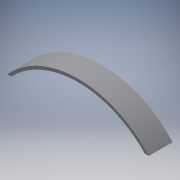
# Autodesk Inventor part: bumper
Saved by Autodesk Inventor 2016 (Build 200138000, 138)
## iProperties
Created: 2015-09-30
Part Number: bumper
Material: Generic
Document SubType Name: Modeling
Designer: Jesse Stevenson
Density: 1 g/cm^3
Appearance: Default
Author: Jesse Stevenson
Autodesk Inventor part; units mm, degrees
ref_plane "YZ Plane" through (0, 0, 0) normal (1, 0, 0) x (0, 1, 0)
ref_plane "XZ Plane" through (0, 0, 0) normal (0, 1, 0) x (-1, 0, 0)
ref_plane "XY Plane" through (0, 0, 0) normal (0, 0, 1) x (1, 0, 0)
sketch "Sketch1" plane through (0, 0, 0) normal (0, 0, 1) x (1, 0, 0)
  arc A0 (0, 0) -> (-150.9369, 0) centre (-75.4685, -68.0226) ccw
  arc A1 (-4.3319, 0) -> (-146.605, 0) centre (-75.4685, -68.0226) ccw
  line L0 (0, 0) -> (-4.3319, 0)
  line L1 (-150.9369, 0) -> (-146.605, 0)
  dimension "d0" = 101.6
  dimension "d1" = 3.175
  constraints: 4 end point, 4 point on circle, 2 centre point, 2 horizontal
  measures "d0" radius of A0
  measures "d1" radial gap between concentric circles of A0 A1
extrude "Extrusion1" add sketch "Sketch1" along normal blind 25.4
ref_plane "Work Plane2" through (-75.4685, -68.0226, 0) normal (1, 0, 0) x (0, 0, 1)
ref_plane "Work Plane1" through (-51.8377, -68.0226, 19.9348) normal (1, 0, 0) x (0, -1, 0)
sketch "Sketch3" plane through (0, 0, 25.4) normal (0, 0, 1) x (1, 0, 0)
  arc A0 (0, 0) -> (-150.9369, 0) centre (-75.4685, -68.0226) ccw construction
  line L0 (-150.9369, 0) -> (-146.605, 0) construction
  arc A1 (-4.3319, 0) -> (-146.605, 0) centre (-75.4685, -68.0226) ccw projected
  line L1 (-4.3319, 0) -> (0, 0) construction
  arc A2 (-4.3319, 0) -> (-146.605, 0) centre (-75.4685, -68.0226) ccw projected
  line L2 (-115.3275, 21.9704) -> (-115.3275, 15.5205)
  line L3 (-115.3275, 15.5205) -> (-106.6482, 15.5205)
  line L4 (-106.6482, 15.5205) -> (-106.6482, 25.3332)
  line L5 (-75.4685, 30.4024) -> (-75.4685, 44.8632) construction
  line L6 (-35.6095, 21.9704) -> (-35.6095, 15.5205)
  line L7 (-35.6095, 15.5205) -> (-44.2887, 15.5205)
  line L8 (-44.2887, 15.5205) -> (-44.2887, 25.3332)
  circle A3 centre (-111.3437, 19.5355) radius 1.7859 projected
  circle A4 centre (-39.5933, 19.5355) radius 1.7859 projected
  line L9 (-44.2887, 25.2167) -> (-44.1786, 25.2964)
  line L10 (-35.6095, 21.8057) -> (-35.7166, 22.0178)
  constraints: 18 end point, 9 point on circle, 4 symmetric about line, 2 perpendicular, 2 point on line, 2 vertical
extrude "Extrusion2" add sketch "Sketch3" against normal blind 3.175 contours L10 L6 L7 L8 L9 A1 | L4 L3 L2 A1
body "Solid1"
